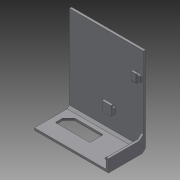
# Autodesk Inventor part: laptop_port_cover
Saved by Autodesk Inventor 2015 SP1 (Build 190203100, 203)
## iProperties
Created: 2014-10-07
Part Number: laptop_port_cover
Material: Generic
Document SubType Name: Modeling
Designer: Drew
Density: 1 g/cm^3
Appearance: Default
Author: Drew
Autodesk Inventor part; units mm, degrees
ref_plane "YZ Plane" through (0, 0, 0) normal (1, 0, 0) x (0, 1, 0)
ref_plane "XZ Plane" through (0, 0, 0) normal (0, 1, 0) x (-1, 0, 0)
ref_plane "XY Plane" through (0, 0, 0) normal (0, 0, 1) x (1, 0, 0)
sketch "Sketch1" plane through (0, 0, 0) normal (0, 1, 0) x (-1, 0, 0)
  line L0 (19.75, 23.5) -> (-19.75, 23.5)
  line L1 (-19.75, 23.5) -> (-19.75, -23.5)
  line L2 (-19.75, -23.5) -> (19.75, -23.5)
  line L3 (19.75, -23.5) -> (19.75, 23.5)
  line L4 (0, -28.9451) -> (0, 30.9067)
  line L5 (30.9717, 0) -> (-30.2589, 0)
  point P0 (0, 0)
  dimension "d0" = 39.5
  dimension "d1" = 47
  constraints: 12 end point, 2 horizontal, 2 parallel, 2 point on line, 1 perpendicular, 1 vertical, 2 other
  measures "d0" distance of L1.end L2.end
  measures "d1" distance of L2.end L0.start
extrude "Extrusion1" add sketch "Sketch1" along normal blind 1.15
sketch "Sketch2" plane through (0, 0, 0) normal (0, 1, 0) x (-1, 0, 0)
  line L0 (-18.6, -22.35) -> (-18.6, -16.9)
  line L1 (-18.6, -16.9) -> (-19.75, -16.9)
  line L2 (-19.75, -16.9) -> (-19.75, -23.5)
  line L3 (-19.75, -23.5) -> (19.75, -23.5)
  line L4 (19.75, -23.5) -> (19.75, -22.35)
  line L5 (19.75, -22.35) -> (-18.6, -22.35)
  line L6 (19.75, -23.5) -> (19.75, 23.5) projected
  point P0 (0, 0)
  point P1 (19.75, -22.925)
  dimension "d7" = 6.6
  dimension "d9" = 1.15
  constraints: 12 end point, 2 parallel, 2 perpendicular, 1 horizontal, 1 midpoint, 1 point on line
  measures "d7" distance of L1.end L2.end
  measures "d9" distance of L3.end L4.end
extrude "Extrusion2" add sketch "Sketch2" against normal blind 18.65
chamfer "Chamfer1" distance 1.15 angle 45 1 edges at (-0.575, 0, -22.35) measured on face at (-0.575, -0.5, -22.35)
chamfer "Chamfer3" distance 1.75 angle 45 1 edges at (0, 1.15, -23.5)
sketch "Sketch3" plane through (19.75, -18.65, -23.5) normal (0, 0, -1) x (-1, 0, 0)
  line L0 (36.4, 8) -> (17.9, 8)
  line L1 (17.9, 8) -> (17.9, 15.2)
  line L2 (17.9, 15.2) -> (33.2, 15.2)
  line L3 (36.4, 12) -> (36.4, 8)
  circle A0 centre (5.5, 5.5) radius 1.35
  line L4 (33.2, 15.2) -> (36.4, 12)
  line L5 (0, 0) -> (0, 18.05) projected
  line L6 (39.5, 0) -> (0, 0) projected
  line L7 (39.5, 0) -> (39.5, 18.05) projected
  point P0 (19.75, 18.65)
  dimension "d19" = 2.7
  dimension "d21" = 135
  dimension "d22" = 135
  dimension "d24" = 18.5
  dimension "d25" = 7.2
  dimension "d34" = 5.5
  dimension "d35" = 5.5
  dimension "d36" = 8
  dimension "d43" = 3.1
  dimension "d47" = 4
  constraints: 10 end point, 2 parallel, 1 centre point, 1 horizontal, 1 perpendicular
  measures "d19" diameter of A0
  measures "d21" angle of L2 L4
  measures "d22" angle of L3 L4
  measures "d24" distance between parallel lines of L1 L3
  measures "d25" distance of L0.end L1.end
  measures "d34" distance from line of A0.centre L5
  measures "d35" distance from line of A0.centre L6
  measures "d36" distance between parallel lines of L0 L6
  measures "d43" distance between parallel lines of L7 L3
  measures "d47" distance of L0.start L3.start
extrude "Extrusion3" cut sketch "Sketch3" against normal blind 1.15
chamfer "Chamfer4" distance 2 angle 45 1 edges at (19.175, 0, -16.9)
chamfer "Chamfer5" distance 1.5 distance2 0.75 1 edges at (15.6, -13.15, -23.5) measured on face at (16.1, -13.15, -23.5)
fillet "Fillet1" radius 0.5 5 edges at (-16.65, -10.65, -22.925) (-16.65, -6.65, -22.925) (-13.45, -3.45, -22.925) (1.85, -10.65, -22.925) (1.85, -3.45, -22.925)
ref_plane "Work Plane1" through (18.5, -18.65, -16.9) normal (1, 0, 0) x (0, 0, -1)
sketch "Sketch5" plane through (18.5, -18.65, -16.9) normal (1, 0, 0) x (0, 0, -1)
  line L0 (-40.4, 18.65) -> (-2, 18.65) projected
  line L1 (-25.55, 18.65) -> (-28.55, 18.65)
  line L2 (-28.55, 18.65) -> (-28.55, 17.15)
  line L3 (-25.55, 16.15) -> (-25.55, 18.65)
  line L4 (-25.55, 16.15) -> (-30.35, 16.15)
  line L5 (-30.35, 16.15) -> (-30.35, 17.15)
  line L6 (-30.35, 17.15) -> (-28.55, 17.15)
  line L7 (5.45, 17.5) -> (5.45, 0) projected
  point P0 (-16.9, 18.65)
  dimension "d52" = 4.8
  dimension "d55" = 1.5
  dimension "d57" = 31
  dimension "d58" = 3
  dimension "d70" = 2.5
  constraints: 12 end point, 2 horizontal, 2 parallel, 2 perpendicular, 1 point on line
  measures "d52" distance between parallel lines of L5 L3
  measures "d55" distance between parallel lines of L0 L6
  measures "d57" distance between parallel lines of L7 L3
  measures "d58" distance between parallel lines of L2 L3
  measures "d70" distance between parallel lines of L4 L0
extrude "Extrusion4" add sketch "Sketch5" against normal blind 3
ref_plane "Work Plane2" through (4.95, -18.65, -16.9) normal (1, 0, 0) x (0, 0, -1)
sketch "Sketch6" plane through (4.95, -18.65, -16.9) normal (1, 0, 0) x (0, 0, -1)
  line L0 (4.3, 18.65) -> (-40.4, 18.65) projected
  line L1 (-4.05, 18.65) -> (-4.05, 16.15)
  line L2 (-4.05, 16.15) -> (-9.05, 16.15)
  line L3 (-9.05, 16.15) -> (-9.05, 17.25)
  line L4 (-9.05, 17.25) -> (-7.05, 17.25)
  line L5 (-7.05, 17.25) -> (-7.05, 18.65)
  line L6 (5.45, 17.5) -> (5.45, 0) projected
  point P0 (-16.9, 18.65)
  dimension "d62" = 5
  dimension "d63" = 2
  dimension "d64" = 2.5
  dimension "d68" = 9.5
  dimension "d69" = 1.4
  constraints: 10 end point, 5 perpendicular, 2 point on line
  measures "d62" distance of L1.end L2.end
  measures "d63" distance of L3.end L4.end
  measures "d64" distance of L1.start L1.end
  measures "d68" distance between parallel lines of L6 L1
  measures "d69" distance between parallel lines of L0 L4
extrude "Extrusion5" add sketch "Sketch6" against normal blind 4.75
fillet "Fillet4" radius 0.5 14 edges at (18.5, -2.5, 11.05) (15.5, -2.5, 11.05) (18.5, -0.75, 11.65) (17, 0, 11.65) (18.5, 0, 10.15) (18.5, -1.25, 8.65) (17, 0, 8.65) (17, -2.5, 8.65) (15.5, -1.25, 8.65) (15.5, 0, 10.15) (15.5, -0.75, 11.65) (15.5, -1.5, 12.55) (18.5, -1.5, 12.55) (17, -1.5, 11.65)
body "Solid1"
